Autodesk Fusion 360 part; units mm, degrees
(part 12 of 15)
  spline S82 degree 5 poles (73.3427, -32.6116) (73.3284, -32.6233) (73.2998, -32.6465) (73.2568, -32.6812) (73.1994, -32.7274) (73.1275, -32.7849) (73.0555, -32.8421) (72.9834, -32.899) (72.9111, -32.9557) (72.8387, -33.012) (72.7662, -33.0681) (72.6935, -33.1239) (72.6207, -33.1794) (72.5478, -33.2347) (72.4747, -33.2896) (72.4015, -33.3442) (72.3282, -33.3986) (72.2547, -33.4527) (72.1811, -33.5064) (72.1073, -33.5599) (72.0334, -33.613) (71.9594, -33.6659) (71.8852, -33.7184) (71.8109, -33.7706) (71.7365, -33.8226) (71.6619, -33.8741) (71.5872, -33.9254) (71.5124, -33.9764) (71.4374, -34.027) (71.3622, -34.0773) (71.287, -34.1272) (71.2115, -34.1768) (71.136, -34.2261) (71.0603, -34.275) (70.9844, -34.3236) (70.9084, -34.3718) (70.8323, -34.4196) (70.756, -34.4671) (70.6795, -34.5142) (70.6029, -34.561) (70.5262, -34.6073) (70.4493, -34.6533) (70.3786, -34.6952) (70.3231, -34.7277) (70.2831, -34.751) (70.2585, -34.7652) (70.2493, -34.7705) knots -1 -1 -1 -1 -1 -1 -0.985714 -0.971429 -0.957143 -0.942857 -0.928571 -0.914286 -0.9 -0.885714 -0.871429 -0.857143 -0.842857 -0.828571 -0.814286 -0.8 -0.785714 -0.771429 -0.757143 -0.742857 -0.728571 -0.714286 -0.7 -0.685714 -0.671429 -0.657143 -0.642857 -0.628571 -0.614286 -0.6 -0.585714 -0.571429 -0.557143 -0.542857 -0.528571 -0.514286 -0.5 -0.485714 -0.471429 -0.457143 -0.442857 -0.428571 -0.414286 -0.405839 -0.405839 -0.405839 -0.405839 -0.405839 -0.405839
  arc A82 (70.5753, -36.0477) -> (70.2493, -34.7705) centre (2.0032, -52.8695) ccw
  spline S83 degree 5 poles (70.5753, -36.0477) (70.5859, -36.0479) (70.6143, -36.0487) (70.6606, -36.0499) (70.7248, -36.0519) (70.807, -36.0547) (70.8965, -36.0582) (70.9861, -36.0621) (71.0757, -36.0664) (71.1654, -36.0712) (71.2551, -36.0763) (71.3449, -36.0818) (71.4347, -36.0877) (71.5245, -36.0939) (71.6144, -36.1006) (71.7043, -36.1076) (71.7943, -36.115) (71.8843, -36.1228) (71.9744, -36.1309) (72.0644, -36.1394) (72.1546, -36.1482) (72.2447, -36.1574) (72.3349, -36.167) (72.4251, -36.1768) (72.5153, -36.1871) (72.6056, -36.1976) (72.6959, -36.2085) (72.7862, -36.2198) (72.8766, -36.2314) (72.9669, -36.2433) (73.0573, -36.2555) (73.1478, -36.2681) (73.2382, -36.2809) (73.3287, -36.2941) (73.4191, -36.3077) (73.5096, -36.3215) (73.6002, -36.3356) (73.6907, -36.3501) (73.7813, -36.3649) (73.8718, -36.38) (73.9624, -36.3953) (74.053, -36.411) (74.1437, -36.427) (74.2162, -36.4401) (74.2706, -36.45) (74.3068, -36.4566) (74.325, -36.46) knots 0.405839 0.405839 0.405839 0.405839 0.405839 0.405839 0.414286 0.428571 0.442857 0.457143 0.471429 0.485714 0.5 0.514286 0.528571 0.542857 0.557143 0.571429 0.585714 0.6 0.614286 0.628571 0.642857 0.657143 0.671429 0.685714 0.7 0.714286 0.728571 0.742857 0.757143 0.771429 0.785714 0.8 0.814286 0.828571 0.842857 0.857143 0.871429 0.885714 0.9 0.914286 0.928571 0.942857 0.957143 0.971429 0.985714 1 1 1 1 1 1
  arc A83 (74.6061, -37.7525) -> (74.325, -36.46) centre (2.0032, -52.8695) ccw
  spline S84 degree 5 poles (74.6061, -37.7525) (74.591, -37.7631) (74.5608, -37.7842) (74.5155, -37.8159) (74.4549, -37.8578) (74.3791, -37.91) (74.3032, -37.9619) (74.2272, -38.0136) (74.1511, -38.0649) (74.0749, -38.116) (73.9985, -38.1667) (73.922, -38.2172) (73.8455, -38.2674) (73.7688, -38.3173) (73.692, -38.3669) (73.615, -38.4162) (73.538, -38.4651) (73.4609, -38.5138) (73.3836, -38.5622) (73.3062, -38.6102) (73.2287, -38.658) (73.1511, -38.7054) (73.0734, -38.7525) (72.9956, -38.7993) (72.9176, -38.8458) (72.8396, -38.8919) (72.7614, -38.9377) (72.6831, -38.9832) (72.6047, -39.0284) (72.5261, -39.0732) (72.4475, -39.1176) (72.3687, -39.1617) (72.2898, -39.2055) (72.2108, -39.2489) (72.1317, -39.2919) (72.0525, -39.3346) (71.9731, -39.3769) (71.8936, -39.4188) (71.814, -39.4603) (71.7343, -39.5015) (71.6544, -39.5422) (71.5745, -39.5826) (71.5009, -39.6193) (71.4433, -39.6478) (71.4017, -39.6682) (71.3761, -39.6806) (71.3666, -39.6853) knots -1 -1 -1 -1 -1 -1 -0.985714 -0.971429 -0.957143 -0.942857 -0.928571 -0.914286 -0.9 -0.885714 -0.871429 -0.857143 -0.842857 -0.828571 -0.814286 -0.8 -0.785714 -0.771429 -0.757143 -0.742857 -0.728571 -0.714286 -0.7 -0.685714 -0.671429 -0.657143 -0.642857 -0.628571 -0.614286 -0.6 -0.585714 -0.571429 -0.557143 -0.542857 -0.528571 -0.514286 -0.5 -0.485714 -0.471429 -0.457143 -0.442857 -0.428571 -0.414286 -0.405839 -0.405839 -0.405839 -0.405839 -0.405839 -0.405839
  arc A84 (71.6006, -40.9824) -> (71.3666, -39.6853) centre (2.0032, -52.8695) ccw
  spline S85 degree 5 poles (71.6006, -40.9824) (71.6112, -40.9834) (71.6395, -40.9862) (71.6856, -40.9907) (71.7495, -40.9973) (71.8312, -41.006) (71.9203, -41.0158) (72.0094, -41.0261) (72.0984, -41.0368) (72.1875, -41.0479) (72.2767, -41.0594) (72.3658, -41.0713) (72.455, -41.0836) (72.5441, -41.0963) (72.6333, -41.1093) (72.7225, -41.1227) (72.8117, -41.1365) (72.901, -41.1507) (72.9902, -41.1652) (73.0795, -41.1801) (73.1687, -41.1954) (73.258, -41.211) (73.3472, -41.2269) (73.4365, -41.2432) (73.5258, -41.2599) (73.6151, -41.2768) (73.7044, -41.2942) (73.7936, -41.3118) (73.8829, -41.3298) (73.9722, -41.3481) (74.0615, -41.3668) (74.1508, -41.3858) (74.2401, -41.4051) (74.3294, -41.4247) (74.4187, -41.4446) (74.508, -41.4649) (74.5973, -41.4854) (74.6865, -41.5063) (74.7758, -41.5275) (74.8651, -41.549) (74.9543, -41.5708) (75.0436, -41.5929) (75.1329, -41.6154) (75.2042, -41.6335) (75.2578, -41.6473) (75.2935, -41.6565) (75.3113, -41.6612) knots 0.405839 0.405839 0.405839 0.405839 0.405839 0.405839 0.414286 0.428571 0.442857 0.457143 0.471429 0.485714 0.5 0.514286 0.528571 0.542857 0.557143 0.571429 0.585714 0.6 0.614286 0.628571 0.642857 0.657143 0.671429 0.685714 0.7 0.714286 0.728571 0.742857 0.757143 0.771429 0.785714 0.8 0.814286 0.828571 0.842857 0.857143 0.871429 0.885714 0.9 0.914286 0.928571 0.942857 0.957143 0.971429 0.985714 1 1 1 1 1 1
  arc A85 (75.4996, -42.9705) -> (75.3113, -41.6612) centre (2.0032, -52.8695) ccw
  spline S86 degree 5 poles (75.4996, -42.9705) (75.4838, -42.98) (75.4521, -42.9989) (75.4046, -43.0272) (75.3412, -43.0647) (75.2619, -43.1114) (75.1825, -43.1577) (75.103, -43.2038) (75.0234, -43.2496) (74.9437, -43.2951) (74.8639, -43.3403) (74.7841, -43.3852) (74.7041, -43.4298) (74.6241, -43.4741) (74.5439, -43.518) (74.4637, -43.5617) (74.3833, -43.6051) (74.3029, -43.6481) (74.2224, -43.6909) (74.1418, -43.7333) (74.0611, -43.7754) (73.9803, -43.8172) (73.8994, -43.8586) (73.8185, -43.8997) (73.7374, -43.9405) (73.6562, -43.981) (73.575, -44.0211) (73.4936, -44.0608) (73.4122, -44.1003) (73.3307, -44.1394) (73.2491, -44.1781) (73.1673, -44.2165) (73.0855, -44.2545) (73.0036, -44.2921) (72.9216, -44.3294) (72.8396, -44.3663) (72.7574, -44.4028) (72.6751, -44.439) (72.5927, -44.4747) (72.5103, -44.5101) (72.4277, -44.5451) (72.3451, -44.5796) (72.2691, -44.611) (72.2096, -44.6353) (72.1666, -44.6526) (72.1402, -44.6632) (72.1304, -44.6672) knots -1 -1 -1 -1 -1 -1 -0.985714 -0.971429 -0.957143 -0.942857 -0.928571 -0.914286 -0.9 -0.885714 -0.871429 -0.857143 -0.842857 -0.828571 -0.814286 -0.8 -0.785714 -0.771429 -0.757143 -0.742857 -0.728571 -0.714286 -0.7 -0.685714 -0.671429 -0.657143 -0.642857 -0.628571 -0.614286 -0.6 -0.585714 -0.571429 -0.557143 -0.542857 -0.528571 -0.514286 -0.5 -0.485714 -0.471429 -0.457143 -0.442857 -0.428571 -0.414286 -0.405839 -0.405839 -0.405839 -0.405839 -0.405839 -0.405839
  arc A86 (72.2713, -45.9777) -> (72.1304, -44.6672) centre (2.0032, -52.8695) ccw
  spline S87 degree 5 poles (72.2713, -45.9777) (72.2817, -45.9795) (72.3098, -45.9842) (72.3555, -45.9921) (72.4188, -46.0032) (72.4997, -46.0177) (72.5878, -46.0339) (72.6759, -46.0505) (72.764, -46.0675) (72.8521, -46.0849) (72.9401, -46.1028) (73.0282, -46.121) (73.1163, -46.1396) (73.2043, -46.1586) (73.2923, -46.178) (73.3804, -46.1977) (73.4684, -46.2179) (73.5563, -46.2384) (73.6443, -46.2592) (73.7323, -46.2804) (73.8202, -46.302) (73.9081, -46.3239) (73.996, -46.3462) (74.0839, -46.3688) (74.1718, -46.3918) (74.2596, -46.4151) (74.3474, -46.4387) (74.4352, -46.4627) (74.523, -46.487) (74.6108, -46.5117) (74.6985, -46.5367) (74.7862, -46.562) (74.8739, -46.5876) (74.9616, -46.6135) (75.0492, -46.6398) (75.1368, -46.6664) (75.2244, -46.6932) (75.312, -46.7204) (75.3995, -46.748) (75.487, -46.7758) (75.5745, -46.8039) (75.662, -46.8323) (75.7494, -46.861) (75.8193, -46.8843) (75.8717, -46.9018) (75.9067, -46.9136) (75.9241, -46.9195) knots 0.405839 0.405839 0.405839 0.405839 0.405839 0.405839 0.414286 0.428571 0.442857 0.457143 0.471429 0.485714 0.5 0.514286 0.528571 0.542857 0.557143 0.571429 0.585714 0.6 0.614286 0.628571 0.642857 0.657143 0.671429 0.685714 0.7 0.714286 0.728571 0.742857 0.757143 0.771429 0.785714 0.8 0.814286 0.828571 0.842857 0.857143 0.871429 0.885714 0.9 0.914286 0.928571 0.942857 0.957143 0.971429 0.985714 1 1 1 1 1 1
  arc A87 (76.0185, -48.2389) -> (75.9241, -46.9195) centre (2.0032, -52.8695) ccw
  spline S88 degree 5 poles (76.0185, -48.2389) (76.0021, -48.2472) (75.9691, -48.2638) (75.9197, -48.2887) (75.8538, -48.3216) (75.7714, -48.3625) (75.6889, -48.403) (75.6063, -48.4433) (75.5236, -48.4833) (75.4409, -48.523) (75.3581, -48.5624) (75.2752, -48.6015) (75.1923, -48.6402) (75.1093, -48.6787) (75.0262, -48.7169) (74.9431, -48.7547) (74.8598, -48.7922) (74.7766, -48.8294) (74.6932, -48.8663) (74.6098, -48.9029) (74.5263, -48.9391) (74.4427, -48.975) (74.3591, -49.0106) (74.2754, -49.0458) (74.1916, -49.0807) (74.1078, -49.1153) (74.0239, -49.1495) (73.9399, -49.1834) (73.8558, -49.2169) (73.7717, -49.25) (73.6876, -49.2828) (73.6033, -49.3153) (73.519, -49.3474) (73.4346, -49.3791) (73.3502, -49.4104) (73.2657, -49.4414) (73.1811, -49.4719) (73.0965, -49.5021) (73.0118, -49.5319) (72.927, -49.5613) (72.8421, -49.5903) (72.7572, -49.6189) (72.6792, -49.6447) (72.6181, -49.6647) (72.574, -49.679) (72.547, -49.6877) (72.5369, -49.6909) knots -1 -1 -1 -1 -1 -1 -0.985714 -0.971429 -0.957143 -0.942857 -0.928571 -0.914286 -0.9 -0.885714 -0.871429 -0.857143 -0.842857 -0.828571 -0.814286 -0.8 -0.785714 -0.771429 -0.757143 -0.742857 -0.728571 -0.714286 -0.7 -0.685714 -0.671429 -0.657143 -0.642857 -0.628571 -0.614286 -0.6 -0.585714 -0.571429 -0.557143 -0.542857 -0.528571 -0.514286 -0.5 -0.485714 -0.471429 -0.457143 -0.442857 -0.428571 -0.414286 -0.405839 -0.405839 -0.405839 -0.405839 -0.405839 -0.405839
  arc A88 (72.5839, -51.0082) -> (72.5369, -49.6909) centre (2.0032, -52.8695) ccw
  spline S89 degree 5 poles (72.5839, -51.0082) (72.5942, -51.0107) (72.6218, -51.0174) (72.6668, -51.0285) (72.7292, -51.044) (72.8089, -51.0643) (72.8956, -51.0867) (72.9823, -51.1096) (73.0689, -51.1329) (73.1556, -51.1565) (73.2421, -51.1806) (73.3287, -51.2051) (73.4152, -51.2299) (73.5016, -51.2551) (73.5881, -51.2807) (73.6744, -51.3067) (73.7608, -51.3331) (73.8471, -51.3598) (73.9333, -51.3869) (74.0196, -51.4143) (74.1057, -51.4421) (74.1919, -51.4702) (74.278, -51.4987) (74.364, -51.5276) (74.45, -51.5567) (74.536, -51.5863) (74.6219, -51.6161) (74.7077, -51.6463) (74.7936, -51.6768) (74.8793, -51.7077) (74.9651, -51.7388) (75.0508, -51.7703) (75.1364, -51.8021) (75.222, -51.8343) (75.3075, -51.8667) (75.393, -51.8995) (75.4785, -51.9325) (75.5639, -51.9659) (75.6492, -51.9996) (75.7345, -52.0336) (75.8198, -52.0679) (75.905, -52.1025) (75.9901, -52.1373) (76.0582, -52.1655) (76.1092, -52.1867) (76.1433, -52.201) (76.1603, -52.2081) knots 0.405839 0.405839 0.405839 0.405839 0.405839 0.405839 0.414286 0.428571 0.442857 0.457143 0.471429 0.485714 0.5 0.514286 0.528571 0.542857 0.557143 0.571429 0.585714 0.6 0.614286 0.628571 0.642857 0.657143 0.671429 0.685714 0.7 0.714286 0.728571 0.742857 0.757143 0.771429 0.785714 0.8 0.814286 0.828571 0.842857 0.857143 0.871429 0.885714 0.9 0.914286 0.928571 0.942857 0.957143 0.971429 0.985714 1 1 1 1 1 1
  arc A89 (76.1603, -53.5309) -> (76.1603, -52.2081) centre (2.0032, -52.8695) ccw
  spline S90 degree 5 poles (76.1603, -53.5309) (76.1433, -53.538) (76.1092, -53.5522) (76.0582, -53.5735) (75.9901, -53.6016) (75.905, -53.6365) (75.8198, -53.6711) (75.7345, -53.7054) (75.6492, -53.7394) (75.5639, -53.7731) (75.4785, -53.8064) (75.393, -53.8395) (75.3075, -53.8723) (75.222, -53.9047) (75.1364, -53.9368) (75.0508, -53.9686) (74.9651, -54.0001) (74.8793, -54.0313) (74.7936, -54.0621) (74.7077, -54.0927) (74.6219, -54.1228) (74.536, -54.1527) (74.45, -54.1822) (74.364, -54.2114) (74.278, -54.2402) (74.1919, -54.2687) (74.1057, -54.2969) (74.0196, -54.3247) (73.9333, -54.3521) (73.8471, -54.3792) (73.7608, -54.4059) (73.6744, -54.4322) (73.5881, -54.4582) (73.5016, -54.4838) (73.4152, -54.5091) (73.3287, -54.5339) (73.2421, -54.5584) (73.1556, -54.5824) (73.0689, -54.6061) (72.9823, -54.6294) (72.8956, -54.6522) (72.8089, -54.6747) (72.7292, -54.6949) (72.6668, -54.7105) (72.6218, -54.7216) (72.5942, -54.7283) (72.5839, -54.7308) knots -1 -1 -1 -1 -1 -1 -0.985714 -0.971429 -0.957143 -0.942857 -0.928571 -0.914286 -0.9 -0.885714 -0.871429 -0.857143 -0.842857 -0.828571 -0.814286 -0.8 -0.785714 -0.771429 -0.757143 -0.742857 -0.728571 -0.714286 -0.7 -0.685714 -0.671429 -0.657143 -0.642857 -0.628571 -0.614286 -0.6 -0.585714 -0.571429 -0.557143 -0.542857 -0.528571 -0.514286 -0.5 -0.485714 -0.471429 -0.457143 -0.442857 -0.428571 -0.414286 -0.405839 -0.405839 -0.405839 -0.405839 -0.405839 -0.405839
  arc A90 (72.5369, -56.0481) -> (72.5839, -54.7308) centre (2.0032, -52.8695) ccw
  spline S91 degree 5 poles (72.5369, -56.0481) (72.547, -56.0513) (72.574, -56.06) (72.6181, -56.0743) (72.6792, -56.0942) (72.7572, -56.1201) (72.8421, -56.1487) (72.927, -56.1777) (73.0118, -56.207) (73.0965, -56.2368) (73.1811, -56.267) (73.2657, -56.2976) (73.3502, -56.3285) (73.4346, -56.3599) (73.519, -56.3916) (73.6033, -56.4237) (73.6876, -56.4561) (73.7717, -56.4889) (73.8558, -56.5221) (73.9399, -56.5556) (74.0239, -56.5895) (74.1078, -56.6237) (74.1916, -56.6582) (74.2754, -56.6931) (74.3591, -56.7284) (74.4427, -56.764) (74.5263, -56.7999) (74.6098, -56.8361) (74.6932, -56.8727) (74.7766, -56.9095) (74.8598, -56.9467) (74.9431, -56.9843) (75.0262, -57.0221) (75.1093, -57.0603) (75.1923, -57.0987) (75.2752, -57.1375) (75.3581, -57.1766) (75.4409, -57.216) (75.5236, -57.2556) (75.6063, -57.2956) (75.6889, -57.3359) (75.7714, -57.3765) (75.8538, -57.4174) (75.9197, -57.4503) (75.9691, -57.4751) (76.0021, -57.4918) (76.0185, -57.5001) knots 0.405839 0.405839 0.405839 0.405839 0.405839 0.405839 0.414286 0.428571 0.442857 0.457143 0.471429 0.485714 0.5 0.514286 0.528571 0.542857 0.557143 0.571429 0.585714 0.6 0.614286 0.628571 0.642857 0.657143 0.671429 0.685714 0.7 0.714286 0.728571 0.742857 0.757143 0.771429 0.785714 0.8 0.814286 0.828571 0.842857 0.857143 0.871429 0.885714 0.9 0.914286 0.928571 0.942857 0.957143 0.971429 0.985714 1 1 1 1 1 1
  arc A91 (75.9241, -58.8195) -> (76.0185, -57.5001) centre (2.0032, -52.8695) ccw
  spline S92 degree 5 poles (75.9241, -58.8195) (75.9067, -58.8254) (75.8717, -58.8371) (75.8193, -58.8547) (75.7494, -58.8779) (75.662, -58.9066) (75.5745, -58.9351) (75.487, -58.9632) (75.3995, -58.991) (75.312, -59.0185) (75.2244, -59.0457) (75.1368, -59.0726) (75.0492, -59.0992) (74.9616, -59.1254) (74.8739, -59.1514) (74.7862, -59.177) (74.6985, -59.2023) (74.6108, -59.2273) (74.523, -59.2519) (74.4352, -59.2762) (74.3474, -59.3002) (74.2596, -59.3239) (74.1718, -59.3472) (74.0839, -59.3701) (73.996, -59.3928) (73.9081, -59.415) (73.8202, -59.437) (73.7323, -59.4585) (73.6443, -59.4798) (73.5563, -59.5006) (73.4684, -59.5211) (73.3804, -59.5412) (73.2923, -59.561) (73.2043, -59.5804) (73.1163, -59.5994) (73.0282, -59.618) (72.9401, -59.6362) (72.8521, -59.654) (72.764, -59.6715) (72.6759, -59.6885) (72.5878, -59.7051) (72.4997, -59.7213) (72.4188, -59.7358) (72.3555, -59.7469) (72.3098, -59.7547) (72.2817, -59.7595) (72.2713, -59.7612) knots -1 -1 -1 -1 -1 -1 -0.985714 -0.971429 -0.957143 -0.942857 -0.928571 -0.914286 -0.9 -0.885714 -0.871429 -0.857143 -0.842857 -0.828571 -0.814286 -0.8 -0.785714 -0.771429 -0.757143 -0.742857 -0.728571 -0.714286 -0.7 -0.685714 -0.671429 -0.657143 -0.642857 -0.628571 -0.614286 -0.6 -0.585714 -0.571429 -0.557143 -0.542857 -0.528571 -0.514286 -0.5 -0.485714 -0.471429 -0.457143 -0.442857 -0.428571 -0.414286 -0.405839 -0.405839 -0.405839 -0.405839 -0.405839 -0.405839
  arc A92 (72.1304, -61.0718) -> (72.2713, -59.7612) centre (2.0032, -52.8695) ccw
  spline S93 degree 5 poles (72.1304, -61.0718) (72.1402, -61.0757) (72.1666, -61.0863) (72.2096, -61.1037) (72.2691, -61.128) (72.3451, -61.1593) (72.4277, -61.1939) (72.5103, -61.2289) (72.5927, -61.2642) (72.6751, -61.3) (72.7574, -61.3361) (72.8396, -61.3727) (72.9216, -61.4096) (73.0036, -61.4469) (73.0855, -61.4845) (73.1673, -61.5225) (73.2491, -61.5609) (73.3307, -61.5996) (73.4122, -61.6387) (73.4936, -61.6781) (73.575, -61.7179) (73.6562, -61.758) (73.7374, -61.7985) (73.8185, -61.8392) (73.8994, -61.8804) (73.9803, -61.9218) (74.0611, -61.9636) (74.1418, -62.0057) (74.2224, -62.0481) (74.3029, -62.0908) (74.3833, -62.1339) (74.4637, -62.1773) (74.5439, -62.2209) (74.6241, -62.2649) (74.7041, -62.3092) (74.7841, -62.3538) (74.8639, -62.3987) (74.9437, -62.4439) (75.0234, -62.4894) (75.103, -62.5351) (75.1825, -62.5812) (75.2619, -62.6276) (75.3412, -62.6742) (75.4046, -62.7118) (75.4521, -62.7401) (75.4838, -62.759) (75.4996, -62.7685) knots 0.405839 0.405839 0.405839 0.405839 0.405839 0.405839 0.414286 0.428571 0.442857 0.457143 0.471429 0.485714 0.5 0.514286 0.528571 0.542857 0.557143 0.571429 0.585714 0.6 0.614286 0.628571 0.642857 0.657143 0.671429 0.685714 0.7 0.714286 0.728571 0.742857 0.757143 0.771429 0.785714 0.8 0.814286 0.828571 0.842857 0.857143 0.871429 0.885714 0.9 0.914286 0.928571 0.942857 0.957143 0.971429 0.985714 1 1 1 1 1 1
  arc A93 (75.3113, -64.0778) -> (75.4996, -62.7685) centre (2.0032, -52.8695) ccw
  spline S94 degree 5 poles (75.3113, -64.0778) (75.2935, -64.0824) (75.2578, -64.0917) (75.2042, -64.1054) (75.1329, -64.1236) (75.0436, -64.146) (74.9543, -64.1681) (74.8651, -64.1899) (74.7758, -64.2114) (74.6865, -64.2326) (74.5973, -64.2535) (74.508, -64.2741) (74.4187, -64.2943) (74.3294, -64.3143) (74.2401, -64.3339) (74.1508, -64.3532) (74.0615, -64.3722) (73.9722, -64.3908) (73.8829, -64.4092) (73.7936, -64.4271) (73.7044, -64.4448) (73.6151, -64.4621) (73.5258, -64.4791) (73.4365, -64.4958) (73.3472, -64.512) (73.258, -64.528) (73.1687, -64.5436) (73.0795, -64.5588) (72.9902, -64.5737) (72.901, -64.5883) (72.8117, -64.6024) (72.7225, -64.6162) (72.6333, -64.6296) (72.5441, -64.6427) (72.455, -64.6554) (72.3658, -64.6676) (72.2767, -64.6795) (72.1875, -64.691) (72.0984, -64.7021) (72.0094, -64.7128) (71.9203, -64.7231) (71.8312, -64.733) (71.7495, -64.7417) (71.6856, -64.7482) (71.6395, -64.7528) (71.6112, -64.7555) (71.6006, -64.7565) knots -1 -1 -1 -1 -1 -1 -0.985714 -0.971429 -0.957143 -0.942857 -0.928571 -0.914286 -0.9 -0.885714 -0.871429 -0.857143 -0.842857 -0.828571 -0.814286 -0.8 -0.785714 -0.771429 -0.757143 -0.742857 -0.728571 -0.714286 -0.7 -0.685714 -0.671429 -0.657143 -0.642857 -0.628571 -0.614286 -0.6 -0.585714 -0.571429 -0.557143 -0.542857 -0.528571 -0.514286 -0.5 -0.485714 -0.471429 -0.457143 -0.442857 -0.428571 -0.414286 -0.405839 -0.405839 -0.405839 -0.405839 -0.405839 -0.405839
  arc A94 (71.3666, -66.0537) -> (71.6006, -64.7565) centre (2.0032, -52.8695) ccw
  spline S95 degree 5 poles (71.3666, -66.0537) (71.3761, -66.0583) (71.4017, -66.0708) (71.4433, -66.0912) (71.5009, -66.1196) (71.5745, -66.1563) (71.6544, -66.1967) (71.7343, -66.2375) (71.814, -66.2786) (71.8936, -66.3202) (71.9731, -66.3621) (72.0525, -66.4044) (72.1317, -66.4471) (72.2108, -66.4901) (72.2898, -66.5335) (72.3687, -66.5773) (72.4475, -66.6214) (72.5261, -66.6658) (72.6047, -66.7106) (72.6831, -66.7557) (72.7614, -66.8012) (72.8396, -66.847) (72.9176, -66.8932) (72.9956, -66.9396) (73.0734, -66.9864) (73.1511, -67.0335) (73.2287, -67.081) (73.3062, -67.1287) (73.3836, -67.1768) (73.4609, -67.2251) (73.538, -67.2738) (73.615, -67.3228) (73.692, -67.3721) (73.7688, -67.4217) (73.8455, -67.4716) (73.922, -67.5218) (73.9985, -67.5722) (74.0749, -67.623) (74.1511, -67.6741) (74.2272, -67.7254) (74.3032, -67.777) (74.3791, -67.8289) (74.4549, -67.8811) (74.5155, -67.9231) (74.5608, -67.9547) (74.591, -67.9758) (74.6061, -67.9864) knots 0.405839 0.405839 0.405839 0.405839 0.405839 0.405839 0.414286 0.428571 0.442857 0.457143 0.471429 0.485714 0.5 0.514286 0.528571 0.542857 0.557143 0.571429 0.585714 0.6 0.614286 0.628571 0.642857 0.657143 0.671429 0.685714 0.7 0.714286 0.728571 0.742857 0.757143 0.771429 0.785714 0.8 0.814286 0.828571 0.842857 0.857143 0.871429 0.885714 0.9 0.914286 0.928571 0.942857 0.957143 0.971429 0.985714 1 1 1 1 1 1
  arc A95 (74.325, -69.279) -> (74.6061, -67.9864) centre (2.0032, -52.8695) ccw
  spline S96 degree 5 poles (74.325, -69.279) (74.3068, -69.2823) (74.2706, -69.289) (74.2162, -69.2989) (74.1437, -69.3119) (74.053, -69.3279) (73.9624, -69.3436) (73.8718, -69.359) (73.7813, -69.3741) (73.6907, -69.3889) (73.6002, -69.4033) (73.5096, -69.4175) (73.4191, -69.4313) (73.3287, -69.4448) (73.2382, -69.458) (73.1478, -69.4709) (73.0573, -69.4835) (72.9669, -69.4957) (72.8766, -69.5076) (72.7862, -69.5192) (72.6959, -69.5304) (72.6056, -69.5413) (72.5153, -69.5519) (72.4251, -69.5621) (72.3349, -69.572) (72.2447, -69.5815) (72.1546, -69.5907) (72.0644, -69.5996) (71.9744, -69.6081) (71.8843, -69.6162) (71.7943, -69.6239) (71.7043, -69.6313) (71.6144, -69.6384) (71.5245, -69.645) (71.4347, -69.6513) (71.3449, -69.6572) (71.2551, -69.6627) (71.1654, -69.6678) (71.0757, -69.6725) (70.9861, -69.6768) (70.8965, -69.6808) (70.807, -69.6843) (70.7248, -69.6871) (70.6606, -69.689) (70.6143, -69.6903) (70.5859, -69.691) (70.5753, -69.6913) knots -1 -1 -1 -1 -1 -1 -0.985714 -0.971429 -0.957143 -0.942857 -0.928571 -0.914286 -0.9 -0.885714 -0.871429 -0.857143 -0.842857 -0.828571 -0.814286 -0.8 -0.785714 -0.771429 -0.757143 -0.742857 -0.728571 -0.714286 -0.7 -0.685714 -0.671429 -0.657143 -0.642857 -0.628571 -0.614286 -0.6 -0.585714 -0.571429 -0.557143 -0.542857 -0.528571 -0.514286 -0.5 -0.485714 -0.471429 -0.457143 -0.442857 -0.428571 -0.414286 -0.405839 -0.405839 -0.405839 -0.405839 -0.405839 -0.405839
  arc A96 (70.2493, -70.9684) -> (70.5753, -69.6913) centre (2.0032, -52.8695) ccw
  spline S97 degree 5 poles (70.2493, -70.9684) (70.2585, -70.9737) (70.2831, -70.988) (70.3231, -71.0113) (70.3786, -71.0438) (70.4493, -71.0856) (70.5262, -71.1316) (70.6029, -71.178) (70.6795, -71.2247) (70.756, -71.2718) (70.8323, -71.3193) (70.9084, -71.3672) (70.9844, -71.4154) (71.0603, -71.464) (71.136, -71.5129) (71.2115, -71.5621) (71.287, -71.6118) (71.3622, -71.6617) (71.4374, -71.712) (71.5124, -71.7626) (71.5872, -71.8135) (71.6619, -71.8648) (71.7365, -71.9164) (71.8109, -71.9683) (71.8852, -72.0205) (71.9594, -72.0731) (72.0334, -72.1259) (72.1073, -72.1791) (72.1811, -72.2325) (72.2547, -72.2863) (72.3282, -72.3404) (72.4015, -72.3947) (72.4747, -72.4494) (72.5478, -72.5043) (72.6207, -72.5595) (72.6935, -72.615) (72.7662, -72.6709) (72.8387, -72.7269) (72.9111, -72.7833) (72.9834, -72.8399) (73.0555, -72.8969) (73.1275, -72.9541) (73.1994, -73.0115) (73.2568, -73.0577) (73.2998, -73.0925) (73.3284, -73.1157) (73.3427, -73.1273) knots 0.405839 0.405839 0.405839 0.405839 0.405839 0.405839 0.414286 0.428571 0.442857 0.457143 0.471429 0.485714 0.5 0.514286 0.528571 0.542857 0.557143 0.571429 0.585714 0.6 0.614286 0.628571 0.642857 0.657143 0.671429 0.685714 0.7 0.714286 0.728571 0.742857 0.757143 0.771429 0.785714 0.8 0.814286 0.828571 0.842857 0.857143 0.871429 0.885714 0.9 0.914286 0.928571 0.942857 0.957143 0.971429 0.985714 1 1 1 1 1 1
  arc A97 (72.97, -74.3965) -> (73.3427, -73.1273) centre (2.0032, -52.8695) ccw
  spline S98 degree 5 poles (72.97, -74.3965) (72.9517, -74.3986) (72.9151, -74.4026) (72.8601, -74.4087) (72.7869, -74.4165) (72.6953, -74.426) (72.6038, -74.4352) (72.5124, -74.444) (72.421, -74.4526) (72.3296, -74.4609) (72.2382, -74.4689) (72.1469, -74.4765) (72.0557, -74.4839) (71.9645, -74.4909) (71.8733, -74.4976) (71.7822, -74.504) (71.6911, -74.5101) (71.6, -74.5158) (71.509, -74.5213) (71.4181, -74.5264) (71.3272, -74.5311) (71.2364, -74.5356) (71.1456, -74.5397) (71.0548, -74.5434) (70.9641, -74.5469) (70.8735, -74.5499) (70.7829, -74.5527) (70.6924, -74.5551) (70.602, -74.5571) (70.5116, -74.5588) (70.4212, -74.5601) (70.331, -74.5611) (70.2408, -74.5616) (70.1506, -74.5619) (70.0606, -74.5617) (69.9706, -74.5612) (69.8806, -74.5603) (69.7908, -74.559) (69.701, -74.5573) (69.6113, -74.5552) (69.5217, -74.5527) (69.4321, -74.5498) (69.35, -74.5468) (69.2858, -74.5441) (69.2395, -74.5421) (69.2111, -74.5408) (69.2005, -74.5403) knots -1 -1 -1 -1 -1 -1 -0.985714 -0.971429 -0.957143 -0.942857 -0.928571 -0.914286 -0.9 -0.885714 -0.871429 -0.857143 -0.842857 -0.828571 -0.814286 -0.8 -0.785714 -0.771429 -0.757143 -0.742857 -0.728571 -0.714286 -0.7 -0.685714 -0.671429 -0.657143 -0.642857 -0.628571 -0.614286 -0.6 -0.585714 -0.571429 -0.557143 -0.542857 -0.528571 -0.514286 -0.5 -0.485714 -0.471429 -0.457143 -0.442857 -0.428571 -0.414286 -0.405839 -0.405839 -0.405839 -0.405839 -0.405839 -0.405839
  arc A98 (68.7843, -75.791) -> (69.2005, -74.5403) centre (2.0032, -52.8695) ccw
  spline S99 degree 5 poles (68.7843, -75.791) (68.793, -75.7969) (68.8166, -75.8129) (68.8548, -75.839) (68.9078, -75.8753) (68.9754, -75.9221) (69.0488, -75.9735) (69.1221, -76.0252) (69.1951, -76.0773) (69.268, -76.1297) (69.3407, -76.1825) (69.4132, -76.2357) (69.4856, -76.2892) (69.5578, -76.3431) (69.6298, -76.3973) (69.7017, -76.4518) (69.7734, -76.5066) (69.8449, -76.5618) (69.9163, -76.6174) (69.9874, -76.6732) (70.0585, -76.7293) (70.1293, -76.7858) (70.2, -76.8426) (70.2706, -76.8997) (70.341, -76.9571) (70.4112, -77.0148) (70.4813, -77.0728) (70.5512, -77.131) (70.6209, -77.1896) (70.6905, -77.2485) (70.7599, -77.3077) (70.8292, -77.3671) (70.8983, -77.4269) (70.9673, -77.4869) (71.0361, -77.5472) (71.1048, -77.6077) (71.1733, -77.6686) (71.2416, -77.7297) (71.3098, -77.7911) (71.3779, -77.8527) (71.4458, -77.9146) (71.5135, -77.9768) (71.5811, -78.0393) (71.635, -78.0894) (71.6754, -78.1272) (71.7023, -78.1524) (71.7158, -78.165) knots 0.405839 0.405839 0.405839 0.405839 0.405839 0.405839 0.414286 0.428571 0.442857 0.457143 0.471429 0.485714 0.5 0.514286 0.528571 0.542857 0.557143 0.571429 0.585714 0.6 0.614286 0.628571 0.642857 0.657143 0.671429 0.685714 0.7 0.714286 0.728571 0.742857 0.757143 0.771429 0.785714 0.8 0.814286 0.828571 0.842857 0.857143 0.871429 0.885714 0.9 0.914286 0.928571 0.942857 0.957143 0.971429 0.985714 1 1 1 1 1 1
  arc A99 (71.2535, -79.4044) -> (71.7158, -78.165) centre (2.0032, -52.8695) ccw
  spline S100 degree 5 poles (71.2535, -79.4044) (71.2351, -79.4051) (71.1982, -79.4066) (71.143, -79.4086) (71.0694, -79.4112) (70.9774, -79.4142) (70.8855, -79.4168) (70.7936, -79.4191) (70.7018, -79.4212) (70.6101, -79.4229) (70.5184, -79.4243) (70.4268, -79.4255) (70.3352, -79.4263) (70.2438, -79.4268) (70.1523, -79.427) (70.061, -79.4268) (69.9697, -79.4264) (69.8785, -79.4257) (69.7873, -79.4246) (69.6962, -79.4232) (69.6052, -79.4214) (69.5143, -79.4194) (69.4235, -79.417) (69.3327, -79.4143) (69.242, -79.4112) (69.1514, -79.4078) (69.0608, -79.4041) (68.9704, -79.4) (68.88, -79.3956) (68.7897, -79.3908) (68.6995, -79.3857) (68.6094, -79.3802) (68.5194, -79.3744) (68.4295, -79.3682) (68.3397, -79.3616) (68.2499, -79.3547) (68.1603, -79.3473) (68.0708, -79.3396) (67.9813, -79.3315) (67.892, -79.3231) (67.8028, -79.3142) (67.7137, -79.3049) (67.632, -79.296) (67.5681, -79.2888) (67.5221, -79.2835) (67.4938, -79.2801) (67.4833, -79.2789) knots -1 -1 -1 -1 -1 -1 -0.985714 -0.971429 -0.957143 -0.942857 -0.928571 -0.914286 -0.9 -0.885714 -0.871429 -0.857143 -0.842857 -0.828571 -0.814286 -0.8 -0.785714 -0.771429 -0.757143 -0.742857 -0.728571 -0.714286 -0.7 -0.685714 -0.671429 -0.657143 -0.642857 -0.628571 -0.614286 -0.6 -0.585714 -0.571429 -0.557143 -0.542857 -0.528571 -0.514286 -0.5 -0.485714 -0.471429 -0.457143 -0.442857 -0.428571 -0.414286 -0.405839 -0.405839 -0.405839 -0.405839 -0.405839 -0.405839
  arc A100 (66.9789, -80.4967) -> (67.4833, -79.2789) centre (2.0032, -52.8695) ccw
  spline S101 degree 5 poles (66.9789, -80.4967) (66.9872, -80.5032) (67.0096, -80.5208) (67.0459, -80.5496) (67.0961, -80.5896) (67.1602, -80.6411) (67.2298, -80.6976) (67.2991, -80.7544) (67.3683, -80.8116) (67.4372, -80.8691) (67.506, -80.9269) (67.5746, -80.9851) (67.6429, -81.0437) (67.7111, -81.1025) (67.7791, -81.1617) (67.8469, -81.2213) (67.9144, -81.2811) (67.9818, -81.3412) (68.0491, -81.4017) (68.1161, -81.4625) (68.1829, -81.5236) (68.2496, -81.5849) (68.3161, -81.6466) (68.3824, -81.7086) (68.4485, -81.7709) (68.5144, -81.8334) (68.5801, -81.8963) (68.6457, -81.9594) (68.7111, -82.0228) (68.7763, -82.0865) (68.8414, -82.1505) (68.9062, -82.2147) (68.9709, -82.2792) (69.0354, -82.344) (69.0997, -82.409) (69.1639, -82.4743) (69.2279, -82.5399) (69.2917, -82.6058) (69.3553, -82.6719) (69.4188, -82.7382) (69.4821, -82.8048) (69.5453, -82.8717) (69.6082, -82.9388) (69.6585, -82.9927) (69.6961, -83.0332) (69.7211, -83.0603) (69.7336, -83.0738) knots 0.405839 0.405839 0.405839 0.405839 0.405839 0.405839 0.414286 0.428571 0.442857 0.457143 0.471429 0.485714 0.5 0.514286 0.528571 0.542857 0.557143 0.571429 0.585714 0.6 0.614286 0.628571 0.642857 0.657143 0.671429 0.685714 0.7 0.714286 0.728571 0.742857 0.757143 0.771429 0.785714 0.8 0.814286 0.828571 0.842857 0.857143 0.871429 0.885714 0.9 0.914286 0.928571 0.942857 0.957143 0.971429 0.985714 1 1 1 1 1 1
  arc A101 (69.1841, -84.2771) -> (69.7336, -83.0738) centre (2.0032, -52.8695) ccw
  spline S102 degree 5 poles (69.1841, -84.2771) (69.1657, -84.2765) (69.1288, -84.2753) (69.0736, -84.2734) (68.9999, -84.2707) (68.908, -84.2671) (68.8161, -84.2632) (68.7243, -84.2589) (68.6326, -84.2544) (68.541, -84.2496) (68.4494, -84.2445) (68.358, -84.2391) (68.2666, -84.2334) (68.1753, -84.2273) (68.0841, -84.221) (67.993, -84.2144) (67.902, -84.2074) (67.811, -84.2002) (67.7202, -84.1926) (67.6295, -84.1847) (67.5388, -84.1765) (67.4483, -84.1679) (67.3578, -84.1591) (67.2675, -84.1499) (67.1772, -84.1404) (67.0871, -84.1305) (66.997, -84.1203) (66.9071, -84.1098) (66.8173, -84.099) (66.7276, -84.0878) (66.638, -84.0762) (66.5485, -84.0643) (66.4591, -84.0521) (66.3698, -84.0395) (66.2807, -84.0265) (66.1917, -84.0132) (66.1028, -83.9995) (66.0141, -83.9854) (65.9254, -83.9709) (65.837, -83.9561) (65.7486, -83.9409) (65.6604, -83.9253) (65.5795, -83.9106) (65.5163, -83.8988) (65.4708, -83.8902) (65.4429, -83.8849) (65.4325, -83.8829) knots -1 -1 -1 -1 -1 -1 -0.985714 -0.971429 -0.957143 -0.942857 -0.928571 -0.914286 -0.9 -0.885714 -0.871429 -0.857143 -0.842857 -0.828571 -0.814286 -0.8 -0.785714 -0.771429 -0.757143 -0.742857 -0.728571 -0.714286 -0.7 -0.685714 -0.671429 -0.657143 -0.642857 -0.628571 -0.614286 -0.6 -0.585714 -0.571429 -0.557143 -0.542857 -0.528571 -0.514286 -0.5 -0.485714 -0.471429 -0.457143 -0.442857 -0.428571 -0.414286 -0.405839 -0.405839 -0.405839 -0.405839 -0.405839 -0.405839
  arc A102 (64.8425, -85.0616) -> (65.4325, -83.8829) centre (2.0032, -52.8695) ccw
  spline S103 degree 5 poles (64.8425, -85.0616) (64.8503, -85.0687) (64.8713, -85.0879) (64.9055, -85.1191) (64.9528, -85.1627) (65.013, -85.2186) (65.0783, -85.2799) (65.1435, -85.3415) (65.2084, -85.4035) (65.2731, -85.4657) (65.3375, -85.5284) (65.4017, -85.5913) (65.4658, -85.6546) (65.5296, -85.7181) (65.5931, -85.782) (65.6565, -85.8462) (65.7197, -85.9108) (65.7826, -85.9756) (65.8453, -86.0407) (65.9078, -86.1061) (65.9702, -86.1718) (66.0323, -86.2377) (66.0942, -86.304) (66.1559, -86.3705) (66.2174, -86.4374) (66.2787, -86.5045) (66.3398, -86.5718) (66.4007, -86.6395) (66.4614, -86.7074) (66.5219, -86.7756) (66.5822, -86.844) (66.6423, -86.9127) (66.7022, -86.9817) (66.7619, -87.0509) (66.8215, -87.1204) (66.8808, -87.1901) (66.9399, -87.2601) (66.9989, -87.3303) (67.0577, -87.4008) (67.1162, -87.4715) (67.1746, -87.5424) (67.2328, -87.6136) (67.2908, -87.6851) (67.3371, -87.7424) (67.3717, -87.7855) (67.3948, -87.8143) (67.4063, -87.8287) knots 0.405839 0.405839 0.405839 0.405839 0.405839 0.405839 0.414286 0.428571 0.442857 0.457143 0.471429 0.485714 0.5 0.514286 0.528571 0.542857 0.557143 0.571429 0.585714 0.6 0.614286 0.628571 0.642857 0.657143 0.671429 0.685714 0.7 0.714286 0.728571 0.742857 0.757143 0.771429 0.785714 0.8 0.814286 0.828571 0.842857 0.857143 0.871429 0.885714 0.9 0.914286 0.928571 0.942857 0.957143 0.971429 0.985714 1 1 1 1 1 1
  arc A103 (66.7723, -88.9897) -> (67.4063, -87.8287) centre (2.0032, -52.8695) ccw
  spline S104 degree 5 poles (66.7723, -88.9897) (66.754, -88.9878) (66.7173, -88.9839) (66.6623, -88.9781) (66.5891, -88.9702) (66.4976, -88.96) (66.4063, -88.9496) (66.315, -88.9388) (66.2239, -88.9277) (66.1328, -88.9164) (66.0419, -88.9048) (65.951, -88.8928) (65.8603, -88.8806) (65.7697, -88.8681) (65.6791, -88.8553) (65.5887, -88.8422) (65.4984, -88.8287) (65.4083, -88.815) (65.3182, -88.801) (65.2282, -88.7866) (65.1384, -88.772) (65.0487, -88.757) (64.9591, -88.7417) (64.8697, -88.7261) (64.7803, -88.7102) (64.6911, -88.6939) (64.602, -88.6773) (64.5131, -88.6604) (64.4242, -88.6432) (64.3356, -88.6256) (64.247, -88.6077) (64.1586, -88.5894) (64.0703, -88.5709) (63.9822, -88.5519) (63.8942, -88.5326) (63.8064, -88.513) (63.7187, -88.493) (63.6312, -88.4726) (63.5438, -88.4519) (63.4566, -88.4307) (63.3696, -88.4093) (63.2827, -88.3874) (63.2031, -88.367) (63.1409, -88.3508) (63.0961, -88.3389) (63.0686, -88.3316) (63.0584, -88.3289) knots -1 -1 -1 -1 -1 -1 -0.985714 -0.971429 -0.957143 -0.942857 -0.928571 -0.914286 -0.9 -0.885714 -0.871429 -0.857143 -0.842857 -0.828571 -0.814286 -0.8 -0.785714 -0.771429 -0.757143 -0.742857 -0.728571 -0.714286 -0.7 -0.685714 -0.671429 -0.657143 -0.642857 -0.628571 -0.614286 -0.6 -0.585714 -0.571429 -0.557143 -0.542857 -0.528571 -0.514286 -0.5 -0.485714 -0.471429 -0.457143 -0.442857 -0.428571 -0.414286 -0.405839 -0.405839 -0.405839 -0.405839 -0.405839 -0.405839
  arc A104 (62.3858, -89.4625) -> (63.0584, -88.3289) centre (2.0032, -52.8695) ccw
  spline S105 degree 5 poles (62.3858, -89.4625) (62.3931, -89.4701) (62.4127, -89.4907) (62.4446, -89.5244) (62.4886, -89.5712) (62.5447, -89.6313) (62.6055, -89.697) (62.6661, -89.7631) (62.7264, -89.8296) (62.7865, -89.8963) (62.8463, -89.9634) (62.9059, -90.0307) (62.9652, -90.0984) (63.0243, -90.1664) (63.0832, -90.2346) (63.1418, -90.3032) (63.2002, -90.372) (63.2583, -90.4412) (63.3163, -90.5106) (63.374, -90.5803) (63.4314, -90.6503) (63.4887, -90.7205) (63.5457, -90.791) (63.6025, -90.8618) (63.6591, -90.9328) (63.7154, -91.0041) (63.7715, -91.0757) (63.8275, -91.1475) (63.8832, -91.2196) (63.9386, -91.2919) (63.9939, -91.3645) (64.049, -91.4373) (64.1038, -91.5103) (64.1585, -91.5837) (64.2129, -91.6572) (64.2671, -91.731) (64.3211, -91.805) (64.3749, -91.8792) (64.4285, -91.9537) (64.4819, -92.0284) (64.535, -92.1034) (64.588, -92.1785) (64.6408, -92.2539) (64.6828, -92.3144) (64.7143, -92.3599) (64.7352, -92.3902) (64.7457, -92.4054) knots 0.405839 0.405839 0.405839 0.405839 0.405839 0.405839 0.414286 0.428571 0.442857 0.457143 0.471429 0.485714 0.5 0.514286 0.528571 0.542857 0.557143 0.571429 0.585714 0.6 0.614286 0.628571 0.642857 0.657143 0.671429 0.685714 0.7 0.714286 0.728571 0.742857 0.757143 0.771429 0.785714 0.8 0.814286 0.828571 0.842857 0.857143 0.871429 0.885714 0.9 0.914286 0.928571 0.942857 0.957143 0.971429 0.985714 1 1 1 1 1 1
  arc A105 (64.0305, -93.5182) -> (64.7457, -92.4054) centre (2.0032, -52.8695) ccw
  spline S106 degree 5 poles (64.0305, -93.5182) (64.0124, -93.515) (63.9761, -93.5086) (63.9216, -93.4989) (63.8491, -93.4857) (63.7586, -93.4691) (63.6683, -93.4521) (63.578, -93.4348) (63.4879, -93.4173) (63.3979, -93.3995) (63.308, -93.3814) (63.2182, -93.363) (63.1286, -93.3444) (63.0391, -93.3254) (62.9497, -93.3062) (62.8605, -93.2866) (62.7714, -93.2668) (62.6824, -93.2467) (62.5936, -93.2263) (62.5049, -93.2055) (62.4163, -93.1845) (62.3279, -93.1632) (62.2396, -93.1415) (62.1515, -93.1196) (62.0635, -93.0973) (61.9757, -93.0747) (61.888, -93.0518) (61.8005, -93.0286) (61.7131, -93.0051) (61.6259, -92.9812) (61.5389, -92.9571) (61.452, -92.9325) (61.3653, -92.9077) (61.2787, -92.8825) (61.1924, -92.857) (61.1062, -92.8311) (61.0201, -92.8049) (60.9343, -92.7784) (60.8486, -92.7515) (60.7631, -92.7242) (60.6778, -92.6965) (60.5927, -92.6685) (60.5148, -92.6425) (60.4539, -92.6219) (60.4101, -92.6069) (60.3832, -92.5976) (60.3732, -92.5941) knots -1 -1 -1 -1 -1 -1 -0.985714 -0.971429 -0.957143 -0.942857 -0.928571 -0.914286 -0.9 -0.885714 -0.871429 -0.857143 -0.842857 -0.828571 -0.814286 -0.8 -0.785714 -0.771429 -0.757143 -0.742857 -0.728571 -0.714286 -0.7 -0.685714 -0.671429 -0.657143 -0.642857 -0.628571 -0.614286 -0.6 -0.585714 -0.571429 -0.557143 -0.542857 -0.528571 -0.514286 -0.5 -0.485714 -0.471429 -0.457143 -0.442857 -0.428571 -0.414286 -0.405839 -0.405839 -0.405839 -0.405839 -0.405839 -0.405839
  arc A106 (59.6214, -93.6769) -> (60.3732, -92.5941) centre (2.0032, -52.8695) ccw
  spline S107 degree 5 poles (59.6214, -93.6769) (59.6282, -93.685) (59.6462, -93.707) (59.6756, -93.7428) (59.7162, -93.7926) (59.7679, -93.8566) (59.8238, -93.9265) (59.8795, -93.9968) (59.935, -94.0673) (59.9901, -94.1382) (60.045, -94.2093) (60.0996, -94.2808) (60.154, -94.3525) (60.2081, -94.4245) (60.2619, -94.4968) (60.3155, -94.5694) (60.3688, -94.6422) (60.4219, -94.7153) (60.4747, -94.7887) (60.5273, -94.8623) (60.5797, -94.9362) (60.6317, -95.0104) (60.6836, -95.0848) (60.7352, -95.1594) (60.7866, -95.2343) (60.8377, -95.3095) (60.8886, -95.3849) (60.9392, -95.4605) (60.9896, -95.5363) (61.0398, -95.6124) (61.0898, -95.6888) (61.1395, -95.7653) (61.189, -95.8421) (61.2383, -95.9191) (61.2873, -95.9964) (61.3361, -96.0738) (61.3847, -96.1515) (61.4331, -96.2294) (61.4812, -96.3075) (61.5291, -96.3858) (61.5768, -96.4644) (61.6243, -96.5431) (61.6715, -96.6221) (61.7092, -96.6854) (61.7373, -96.733) (61.756, -96.7648) (61.7653, -96.7807) knots 0.405839 0.405839 0.405839 0.405839 0.405839 0.405839 0.414286 0.428571 0.442857 0.457143 0.471429 0.485714 0.5 0.514286 0.528571 0.542857 0.557143 0.571429 0.585714 0.6 0.614286 0.628571 0.642857 0.657143 0.671429 0.685714 0.7 0.714286 0.728571 0.742857 0.757143 0.771429 0.785714 0.8 0.814286 0.828571 0.842857 0.857143 0.871429 0.885714 0.9 0.914286 0.928571 0.942857 0.957143 0.971429 0.985714 1 1 1 1 1 1
  arc A107 (60.9726, -97.8396) -> (61.7653, -96.7807) centre (2.0032, -52.8695) ccw
  spline S108 degree 5 poles (60.9726, -97.8396) (60.9548, -97.8351) (60.919, -97.8261) (60.8654, -97.8126) (60.794, -97.7943) (60.705, -97.7712) (60.616, -97.7478) (60.5272, -97.7242) (60.4386, -97.7003) (60.3501, -97.6761) (60.2617, -97.6516) (60.1735, -97.6269) (60.0854, -97.6019) (59.9975, -97.5766) (59.9097, -97.551) (59.8221, -97.5252) (59.7346, -97.499) (59.6473, -97.4726) (59.5602, -97.4459) (59.4732, -97.4189) (59.3863, -97.3916) (59.2997, -97.364) (59.2132, -97.3361) (59.1268, -97.3079) (59.0407, -97.2795) (58.9547, -97.2507) (58.8689, -97.2216) (58.7832, -97.1922) (58.6978, -97.1625) (58.6125, -97.1325) (58.5274, -97.1021) (58.4425, -97.0715) (58.3577, -97.0405) (58.2732, -97.0092) (58.1889, -96.9776) (58.1047, -96.9457) (58.0208, -96.9134) (57.9371, -96.8808) (57.8535, -96.8478) (57.7702, -96.8145) (57.6871, -96.7809) (57.6042, -96.7469) (57.5283, -96.7153) (57.4691, -96.6904) (57.4264, -96.6723) (57.4003, -96.6611) (57.3905, -96.657) knots -1 -1 -1 -1 -1 -1 -0.985714 -0.971429 -0.957143 -0.942857 -0.928571 -0.914286 -0.9 -0.885714 -0.871429 -0.857143 -0.842857 -0.828571 -0.814286 -0.8 -0.785714 -0.771429 -0.757143 -0.742857 -0.728571 -0.714286 -0.7 -0.685714 -0.671429 -0.657143 -0.642857 -0.628571 -0.614286 -0.6 -0.585714 -0.571429 -0.557143 -0.542857 -0.528571 -0.514286 -0.5 -0.485714 -0.471429 -0.457143 -0.442857 -0.428571 -0.414286 -0.405839 -0.405839 -0.405839 -0.405839 -0.405839 -0.405839
  arc A108 (56.5635, -97.6833) -> (57.3905, -96.657) centre (2.0032, -52.8695) ccw
  spline S109 degree 5 poles (56.5635, -97.6833) (56.5696, -97.6919) (56.5861, -97.7151) (56.6128, -97.753) (56.6497, -97.8056) (56.6967, -97.873) (56.7476, -97.9468) (56.7981, -98.0208) (56.8484, -98.0952) (56.8983, -98.1698) (56.948, -98.2447) (56.9974, -98.3198) (57.0465, -98.3953) (57.0953, -98.4709) (57.1438, -98.5469) (57.1921, -98.6231) (57.2401, -98.6996) (57.2878, -98.7763) (57.3353, -98.8532) (57.3825, -98.9304) (57.4294, -99.0078) (57.4761, -99.0855) (57.5225, -99.1634) (57.5686, -99.2416) (57.6145, -99.3199) (57.6601, -99.3985) (57.7055, -99.4774) (57.7507, -99.5564) (57.7955, -99.6357) (57.8402, -99.7152) (57.8845, -99.7948) (57.9287, -99.8748) (57.9726, -99.9549) (58.0162, -100.0352) (58.0596, -100.1157) (58.1028, -100.1965) (58.1457, -100.2774) (58.1884, -100.3586) (58.2308, -100.4399) (58.273, -100.5215) (58.315, -100.6032) (58.3567, -100.6852) (58.3982, -100.7673) (58.4313, -100.8331) (58.4559, -100.8826) (58.4723, -100.9157) (58.4805, -100.9322) knots 0.405839 0.405839 0.405839 0.405839 0.405839 0.405839 0.414286 0.428571 0.442857 0.457143 0.471429 0.485714 0.5 0.514286 0.528571 0.542857 0.557143 0.571429 0.585714 0.6 0.614286 0.628571 0.642857 0.657143 0.671429 0.685714 0.7 0.714286 0.728571 0.742857 0.757143 0.771429 0.785714 0.8 0.814286 0.828571 0.842857 0.857143 0.871429 0.885714 0.9 0.914286 0.928571 0.942857 0.957143 0.971429 0.985714 1 1 1 1 1 1
  arc A109 (57.6143, -101.9319) -> (58.4805, -100.9322) centre (2.0032, -52.8695) ccw
  spline S110 degree 5 poles (57.6143, -101.9319) (57.5967, -101.9261) (57.5617, -101.9146) (57.5092, -101.8972) (57.4393, -101.8739) (57.3521, -101.8445) (57.2651, -101.8149) (57.1782, -101.785) (57.0915, -101.7548) (57.0049, -101.7243) (56.9185, -101.6936) (56.8323, -101.6627) (56.7462, -101.6315) (56.6603, -101.6) (56.5746, -101.5682) (56.4891, -101.5361) (56.4037, -101.5038) (56.3185, -101.4712) (56.2335, -101.4384) (56.1486, -101.4052) (56.064, -101.3718) (55.9795, -101.3381) (55.8952, -101.3041) (55.8111, -101.2699) (55.7272, -101.2353) (55.6435, -101.2005) (55.5599, -101.1653) (55.4766, -101.1299) (55.3935, -101.0942) (55.3106, -101.0582) (55.2278, -101.0218) (55.1453, -100.9852) (55.063, -100.9483) (54.9809, -100.911) (54.8991, -100.8735) (54.8174, -100.8356) (54.736, -100.7974) (54.6548, -100.7589) (54.5739, -100.7201) (54.4931, -100.6809) (54.4126, -100.6414) (54.3324, -100.6016) (54.2589, -100.5647) (54.2016, -100.5356) (54.1604, -100.5146) (54.1351, -100.5016) (54.1257, -100.4967) knots -1 -1 -1 -1 -1 -1 -0.985714 -0.971429 -0.957143 -0.942857 -0.928571 -0.914286 -0.9 -0.885714 -0.871429 -0.857143 -0.842857 -0.828571 -0.814286 -0.8 -0.785714 -0.771429 -0.757143 -0.742857 -0.728571 -0.714286 -0.7 -0.685714 -0.671429 -0.657143 -0.642857 -0.628571 -0.614286 -0.6 -0.585714 -0.571429 -0.557143 -0.542857 -0.528571 -0.514286 -0.5 -0.485714 -0.471429 -0.457143 -0.442857 -0.428571 -0.414286 -0.405839 -0.405839 -0.405839 -0.405839 -0.405839 -0.405839
  arc A110 (53.2275, -101.4614) -> (54.1257, -100.4967) centre (2.0032, -52.8695) ccw
  spline S111 degree 5 poles (53.2275, -101.4614) (53.233, -101.4705) (53.2477, -101.4948) (53.2717, -101.5344) (53.3048, -101.5895) (53.3468, -101.6602) (53.3923, -101.7374) (53.4374, -101.8148) (53.4822, -101.8926) (53.5268, -101.9705) (53.571, -102.0488) (53.6149, -102.1273) (53.6585, -102.206) (53.7018, -102.285) (53.7448, -102.3642) (53.7875, -102.4437) (53.8299, -102.5233) (53.872, -102.6033) (53.9139, -102.6834) (53.9554, -102.7638) (53.9967, -102.8444) (54.0377, -102.9252) (54.0784, -103.0062) (54.1189, -103.0874) (54.1591, -103.1689) (54.199, -103.2505) (54.2386, -103.3324) (54.278, -103.4144) (54.3171, -103.4967) (54.356, -103.5792) (54.3945, -103.6618) (54.4329, -103.7447) (54.4709, -103.8277) (54.5087, -103.911) (54.5463, -103.9944) (54.5836, -104.078) (54.6206, -104.1618) (54.6574, -104.2458) (54.6939, -104.33) (54.7302, -104.4143) (54.7662, -104.4988) (54.802, -104.5835) (54.8376, -104.6684) (54.8658, -104.7365) (54.8869, -104.7876) (54.9009, -104.8217) (54.9078, -104.8388) knots 0.405839 0.405839 0.405839 0.405839 0.405839 0.405839 0.414286 0.428571 0.442857 0.457143 0.471429 0.485714 0.5 0.514286 0.528571 0.542857 0.557143 0.571429 0.585714 0.6 0.614286 0.628571 0.642857 0.657143 0.671429 0.685714 0.7 0.714286 0.728571 0.742857 0.757143 0.771429 0.785714 0.8 0.814286 0.828571 0.842857 0.857143 0.871429 0.885714 0.9 0.914286 0.928571 0.942857 0.957143 0.971429 0.985714 1 1 1 1 1 1
  arc A111 (53.9725, -105.7741) -> (54.9078, -104.8388) centre (2.0032, -52.8695) ccw
  spline S112 degree 5 poles (53.9725, -105.7741) (53.9554, -105.7671) (53.9213, -105.7531) (53.8702, -105.7321) (53.8022, -105.7038) (53.7173, -105.6683) (53.6326, -105.6325) (53.548, -105.5965) (53.4637, -105.5602) (53.3795, -105.5236) (53.2955, -105.4869) (53.2117, -105.4498) (53.1281, -105.4125) (53.0447, -105.375) (52.9615, -105.3372) (52.8784, -105.2991) (52.7955, -105.2608) (52.7129, -105.2222) (52.6304, -105.1834) (52.5482, -105.1443) (52.4661, -105.1049) (52.3842, -105.0653) (52.3026, -105.0253) (52.2211, -104.9852) (52.1399, -104.9447) (52.0589, -104.904) (51.9781, -104.863) (51.8975, -104.8217) (51.8171, -104.7801) (51.737, -104.7383) (51.6571, -104.6962) (51.5774, -104.6537) (51.4979, -104.611) (51.4187, -104.568) (51.3397, -104.5247) (51.261, -104.4811) (51.1825, -104.4372) (51.1043, -104.393) (51.0263, -104.3485) (50.9486, -104.3037) (50.8711, -104.2586) (50.7939, -104.2131) (50.7232, -104.1711) (50.6682, -104.138) (50.6285, -104.114) (50.6042, -104.0992) (50.5952, -104.0937) knots -1 -1 -1 -1 -1 -1 -0.985714 -0.971429 -0.957143 -0.942857 -0.928571 -0.914286 -0.9 -0.885714 -0.871429 -0.857143 -0.842857 -0.828571 -0.814286 -0.8 -0.785714 -0.771429 -0.757143 -0.742857 -0.728571 -0.714286 -0.7 -0.685714 -0.671429 -0.657143 -0.642857 -0.628571 -0.614286 -0.6 -0.585714 -0.571429 -0.557143 -0.542857 -0.528571 -0.514286 -0.5 -0.485714 -0.471429 -0.457143 -0.442857 -0.428571 -0.414286 -0.405839 -0.405839 -0.405839 -0.405839 -0.405839 -0.405839
  arc A112 (49.6305, -104.9919) -> (50.5952, -104.0937) centre (2.0032, -52.8695) ccw
  spline S113 degree 5 poles (49.6305, -104.9919) (49.6353, -105.0013) (49.6483, -105.0266) (49.6694, -105.0679) (49.6985, -105.1252) (49.7353, -105.1987) (49.7752, -105.2789) (49.8147, -105.3594) (49.8538, -105.4401) (49.8927, -105.5211) (49.9312, -105.6023) (49.9693, -105.6837) (50.0072, -105.7653) (50.0448, -105.8472) (50.082, -105.9293) (50.1189, -106.0116) (50.1556, -106.0941) (50.1919, -106.1768) (50.2279, -106.2597) (50.2636, -106.3429) (50.2991, -106.4262) (50.3342, -106.5097) (50.3691, -106.5934) (50.4036, -106.6774) (50.4379, -106.7615) (50.4719, -106.8457) (50.5056, -106.9302) (50.539, -107.0149) (50.5721, -107.0997) (50.605, -107.1848) (50.6376, -107.27) (50.6699, -107.3553) (50.7019, -107.4409) (50.7337, -107.5266) (50.7652, -107.6125) (50.7964, -107.6986) (50.8274, -107.7848) (50.8581, -107.8712) (50.8885, -107.9578) (50.9187, -108.0445) (50.9486, -108.1314) (50.9783, -108.2184) (51.0077, -108.3056) (51.031, -108.3755) (51.0483, -108.428) (51.0598, -108.463) (51.0656, -108.4805) knots 0.405839 0.405839 0.405839 0.405839 0.405839 0.405839 0.414286 0.428571 0.442857 0.457143 0.471429 0.485714 0.5 0.514286 0.528571 0.542857 0.557143 0.571429 0.585714 0.6 0.614286 0.628571 0.642857 0.657143 0.671429 0.685714 0.7 0.714286 0.728571 0.742857 0.757143 0.771429 0.785714 0.8 0.814286 0.828571 0.842857 0.857143 0.871429 0.885714 0.9 0.914286 0.928571 0.942857 0.957143 0.971429 0.985714 1 1 1 1 1 1
  arc A113 (50.0659, -109.3468) -> (51.0656, -108.4805) centre (2.0032, -52.8695) ccw
  spline S114 degree 5 poles (50.0659, -109.3468) (50.0494, -109.3386) (50.0164, -109.3222) (49.9669, -109.2975) (49.901, -109.2645) (49.8189, -109.223) (49.737, -109.1813) (49.6552, -109.1393) (49.5737, -109.0971) (49.4923, -109.0546) (49.4112, -109.012) (49.3302, -108.969) (49.2495, -108.9259) (49.1689, -108.8825) (49.0886, -108.8388) (49.0085, -108.7949) (48.9286, -108.7508) (48.8489, -108.7064) (48.7694, -108.6618) (48.6901, -108.6169) (48.6111, -108.5718) (48.5323, -108.5264) (48.4537, -108.4808) (48.3753, -108.4349) (48.2972, -108.3887) (48.2193, -108.3423) (48.1416, -108.2957) (48.0641, -108.2487) (47.987, -108.2016) (47.91, -108.1541) (47.8333, -108.1064) (47.7568, -108.0584) (47.6806, -108.0101) (47.6047, -107.9616) (47.529, -107.9127) (47.4536, -107.8636) (47.3784, -107.8142) (47.3035, -107.7646) (47.2289, -107.7146) (47.1546, -107.6644) (47.0805, -107.6138) (47.0068, -107.563) (46.9393, -107.516) (46.8867, -107.4791) (46.8489, -107.4523) (46.8257, -107.4359) (46.8171, -107.4297) knots -1 -1 -1 -1 -1 -1 -0.985714 -0.971429 -0.957143 -0.942857 -0.928571 -0.914286 -0.9 -0.885714 -0.871429 -0.857143 -0.842857 -0.828571 -0.814286 -0.8 -0.785714 -0.771429 -0.757143 -0.742857 -0.728571 -0.714286 -0.7 -0.685714 -0.671429 -0.657143 -0.642857 -0.628571 -0.614286 -0.6 -0.585714 -0.571429 -0.557143 -0.542857 -0.528571 -0.514286 -0.5 -0.485714 -0.471429 -0.457143 -0.442857 -0.428571 -0.414286 -0.405839 -0.405839 -0.405839 -0.405839 -0.405839 -0.405839
  arc A114 (45.7907, -108.2568) -> (46.8171, -107.4297) centre (2.0032, -52.8695) ccw